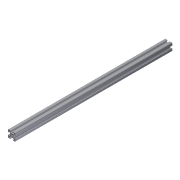
# Autodesk Inventor part: short side
Saved by Autodesk Inventor 2011 (Build 150239000, 239)
## iProperties
Created: 2013-10-03
Part Number: short side
Document SubType Name: Modeling
Designer: Family Room
Density: 1 g/cm^3
Author: Family Room
Autodesk Inventor part; units mm, degrees
ref_plane "YZ Plane" through (0, 0, 0) normal (1, 0, 0) x (0, 1, 0)
ref_plane "XZ Plane" through (0, 0, 0) normal (0, 1, 0) x (-1, 0, 0)
ref_plane "XY Plane" through (0, 0, 0) normal (0, 0, 1) x (1, 0, 0)
sketch "Sketch1" plane through (0, 0, 0) normal (0, 0, 1) x (1, 0, 0)
  line L0 (11.2616, 7.5565) -> (11.8104, 7.0077)
  line L1 (11.8104, 7.0077) -> (12.9923, 8.1896)
  line L2 (12.9923, 8.1896) -> (12.4435, 8.7384)
  arc A0 (12.4435, 8.7384) -> (12.4435, 11.2616) centre (10, 10) ccw
  line L3 (12.4435, 11.2616) -> (12.9923, 11.8104)
  line L4 (12.9923, 11.8104) -> (11.8104, 12.9923)
  line L5 (11.8104, 12.9923) -> (11.2616, 12.4435)
  arc A1 (11.2616, 12.4435) -> (8.7384, 12.4435) centre (10, 10) ccw
  line L6 (8.7384, 12.4435) -> (8.1896, 12.9923)
  line L7 (8.1896, 12.9923) -> (7.0077, 11.8104)
  line L8 (7.0077, 11.8104) -> (7.5565, 11.2616)
  arc A2 (7.5565, 11.2616) -> (7.5565, 8.7384) centre (10, 10) ccw
  line L9 (7.5565, 8.7384) -> (7.0077, 8.1896)
  line L10 (7.0077, 8.1896) -> (8.1896, 7.0077)
  line L11 (8.1896, 7.0077) -> (8.7384, 7.5565)
  arc A3 (8.7384, 7.5565) -> (11.2616, 7.5565) centre (10, 10) ccw
  line L12 (13.4545, 0) -> (13.4545, 0.5)
  line L13 (13.4545, 0.5) -> (13, 0.5)
  line L14 (13, 0.5) -> (13, 1.5)
  line L15 (13, 1.5) -> (15.9091, 1.5)
  line L16 (15.9091, 1.5) -> (15.9091, 3)
  line L17 (15.9091, 3) -> (13.4545, 5.4545)
  line L18 (13.4545, 5.4545) -> (10.8302, 5.4545)
  arc A4 (10.8302, 5.4545) -> (9.1698, 5.4545) centre (10, 5.1837) ccw
  line L19 (9.1698, 5.4545) -> (6.6667, 5.4545)
  line L20 (6.6667, 5.4545) -> (4, 2.9545)
  line L21 (4, 2.9545) -> (4, 1.5909)
  line L22 (4, 1.5909) -> (7, 1.5909)
  line L23 (7, 1.5909) -> (7, 0.4545)
  line L24 (7, 0.4545) -> (6.6667, 0.4545)
  line L25 (6.6667, 0.4545) -> (6.6667, 0)
  line L26 (6.6667, 0) -> (1.5043, 0)
  arc A5 (0, 1.5043) -> (1.5043, 0) centre (1.5043, 1.5043) ccw
  line L27 (0, 1.5043) -> (0, 6.5455)
  line L28 (0, 6.5455) -> (0.5, 6.5455)
  line L29 (0.5, 6.5455) -> (0.5, 7)
  line L30 (0.5, 7) -> (1.5, 7)
  line L31 (1.5, 7) -> (1.5, 4.0909)
  line L32 (1.5, 4.0909) -> (3, 4.0909)
  line L33 (3, 4.0909) -> (5.4545, 6.5455)
  line L34 (5.4545, 6.5455) -> (5.4545, 9.1698)
  arc A6 (5.4545, 9.1698) -> (5.4545, 10.8302) centre (5.1837, 10) ccw
  line L35 (5.4545, 10.8302) -> (5.4545, 13.3333)
  line L36 (5.4545, 13.3333) -> (2.9545, 16)
  line L37 (2.9545, 16) -> (1.5909, 16)
  line L38 (1.5909, 16) -> (1.5909, 13)
  line L39 (1.5909, 13) -> (0.4545, 13)
  line L40 (0.4545, 13) -> (0.4545, 13.3333)
  line L41 (0.4545, 13.3333) -> (0, 13.3333)
  line L42 (0, 13.3333) -> (0, 18.4957)
  arc A7 (1.5043, 20) -> (0, 18.4957) centre (1.5043, 18.4957) ccw
  line L43 (1.5043, 20) -> (6.5455, 20)
  line L44 (6.5455, 20) -> (6.5455, 19.5)
  line L45 (6.5455, 19.5) -> (7, 19.5)
  line L46 (7, 19.5) -> (7, 18.5)
  line L47 (7, 18.5) -> (4.0909, 18.5)
  line L48 (4.0909, 18.5) -> (4.0909, 17)
  line L49 (4.0909, 17) -> (6.5455, 14.5455)
  line L50 (6.5455, 14.5455) -> (9.1698, 14.5455)
  arc A8 (9.1698, 14.5455) -> (10.8302, 14.5455) centre (10, 14.8163) ccw
  line L51 (10.8302, 14.5455) -> (13.3333, 14.5455)
  line L52 (13.3333, 14.5455) -> (16, 17.0455)
  line L53 (16, 17.0455) -> (16, 18.4091)
  line L54 (16, 18.4091) -> (13, 18.4091)
  line L55 (13, 18.4091) -> (13, 19.5455)
  line L56 (13, 19.5455) -> (13.3333, 19.5455)
  line L57 (13.3333, 19.5455) -> (13.3333, 20)
  line L58 (13.3333, 20) -> (18.4957, 20)
  arc A9 (20, 18.4957) -> (18.4957, 20) centre (18.4957, 18.4957) ccw
  line L59 (20, 18.4957) -> (20, 13.4545)
  line L60 (20, 13.4545) -> (19.5, 13.4545)
  line L61 (19.5, 13.4545) -> (19.5, 13)
  line L62 (19.5, 13) -> (18.5, 13)
  line L63 (18.5, 13) -> (18.5, 15.9091)
  line L64 (18.5, 15.9091) -> (17, 15.9091)
  line L65 (17, 15.9091) -> (14.5455, 13.4545)
  line L66 (14.5455, 13.4545) -> (14.5455, 10.8302)
  arc A10 (14.5455, 10.8302) -> (14.5455, 9.1698) centre (14.8163, 10) ccw
  line L67 (14.5455, 9.1698) -> (14.5455, 6.6667)
  line L68 (14.5455, 6.6667) -> (17.0455, 4)
  line L69 (17.0455, 4) -> (18.4091, 4)
  line L70 (18.4091, 4) -> (18.4091, 7)
  line L71 (18.4091, 7) -> (19.5455, 7)
  line L72 (19.5455, 7) -> (19.5455, 6.6667)
  line L73 (19.5455, 6.6667) -> (20, 6.6667)
  line L74 (20, 6.6667) -> (20, 1.5043)
  arc A11 (18.4957, 0) -> (20, 1.5043) centre (18.4957, 1.5043) ccw
  line L75 (18.4957, 0) -> (13.4545, 0)
  point P0 (0, 0)
  point P1 (0.4406, 0.4406)
  point P2 (10, 0)
  point P3 (10, 0)
  point P4 (10, 0)
  point P5 (19.5594, 0.4406)
  point P6 (0, 10)
  point P7 (0, 10)
  point P8 (0, 10)
  point P9 (10, 10)
  point P10 (20, 10)
  point P11 (20, 10)
  point P12 (20, 10)
  point P13 (0.4406, 19.5594)
  point P14 (10, 20)
  point P15 (10, 20)
  point P16 (10, 20)
  point P17 (19.5594, 19.5594)
  constraints: 152 end point, 28 point on circle, 12 centre point
extrude "Extrusion1" add sketch "Sketch1" along normal mid plane 424.5
body "Solid1"
